Autodesk Inventor part; units mm, degrees
(part 3 of 3)
sketch "Sketch43" plane through (-2.5, -2.5, 2) normal (0, -1, 0) x (1, 0, 0)
  line L0 (109.4941, -32.48) -> (111.9941, -28.1499)
  line L1 (111.9941, -28.1499) -> (116.9941, -28.1499)
  line L2 (116.9941, -28.1499) -> (119.4941, -32.48)
  line L3 (89.4941, -32.48) -> (91.9941, -28.1499) construction
  line L4 (91.9941, -28.1499) -> (96.9941, -28.1499) construction
  line L5 (96.9941, -28.1499) -> (99.4941, -32.48) construction
  line L6 (119.4941, -32.3134) -> (129.4941, -32.3134) construction
  line L7 (119.4941, -19.65) -> (121.9941, -15.3199)
  line L8 (121.9941, -15.3199) -> (126.9941, -15.3199)
  line L9 (126.9941, -23.9801) -> (121.9941, -23.9801)
  line L10 (121.9941, -23.9801) -> (119.4941, -19.65)
  line L11 (109.4941, -6.3326) -> (111.9941, -2.0025)
  line L12 (111.9941, -10.6628) -> (109.4941, -6.3326)
  line L13 (116.9941, -10.6628) -> (111.9941, -10.6628)
  line L14 (111.9941, -2.0025) -> (116.9941, -2.0025)
  line L15 (119.4941, -6.3326) -> (116.9941, -10.6628)
  line L16 (116.9941, -2.0025) -> (119.4941, -6.3326)
  line L17 (96.9941, -10.6628) -> (91.9941, -10.6628)
  line L18 (91.9941, -10.6628) -> (89.4941, -6.3326)
  line L19 (99.4941, -6.3326) -> (96.9941, -10.6628)
  line L20 (89.4941, -6.3326) -> (91.9941, -2.0025)
  line L21 (91.9941, -2.0025) -> (96.9941, -2.0025)
  line L22 (96.9941, -2.0025) -> (99.4941, -6.3326)
  line L23 (99.4941, -19.65) -> (101.9941, -15.3199)
  line L24 (101.9941, -15.3199) -> (106.9941, -15.3199)
  line L25 (106.9941, -15.3199) -> (109.4941, -19.65)
  line L26 (109.4941, -19.65) -> (106.9941, -23.9801)
  line L27 (106.9941, -23.9801) -> (101.9941, -23.9801)
  line L28 (101.9941, -23.9801) -> (99.4941, -19.65)
  line L29 (69.4941, -32.48) -> (71.9941, -28.1499)
  line L30 (71.9941, -28.1499) -> (76.9941, -28.1499)
  line L31 (76.9941, -28.1499) -> (79.4941, -32.48)
  line L32 (49.4941, -32.48) -> (51.9941, -28.1499)
  line L33 (51.9941, -28.1499) -> (56.9941, -28.1499)
  line L34 (56.9941, -28.1499) -> (59.4941, -32.48)
  line L35 (79.4941, -32.48) -> (89.4941, -32.48) construction
  line L36 (79.4941, -19.65) -> (81.9941, -15.3199)
  line L37 (81.9941, -23.9801) -> (79.4941, -19.65)
  line L38 (81.9941, -15.3199) -> (86.9941, -15.3199)
  line L39 (86.9941, -15.3199) -> (89.4941, -19.65)
  line L40 (89.4941, -19.65) -> (86.9941, -23.9801)
  line L41 (86.9941, -23.9801) -> (81.9941, -23.9801)
  line L42 (69.4941, -19.65) -> (66.9941, -23.9801)
  line L43 (76.9941, -10.6628) -> (71.9941, -10.6628)
  line L44 (66.9941, -15.3199) -> (69.4941, -19.65)
  line L45 (66.9941, -23.9801) -> (61.9941, -23.9801)
  line L46 (61.9941, -23.9801) -> (59.4941, -19.65)
  line L47 (59.4941, -19.65) -> (61.9941, -15.3199)
  line L48 (61.9941, -15.3199) -> (66.9941, -15.3199)
  line L49 (71.9941, -10.6628) -> (69.4941, -6.3326)
  line L50 (71.9941, -2.0025) -> (76.9941, -2.0025)
  line L51 (69.4941, -6.3326) -> (71.9941, -2.0025)
  line L52 (76.9941, -2.0025) -> (79.4941, -6.3326)
  line L53 (79.4941, -6.3326) -> (76.9941, -10.6628)
  line L54 (59.4941, -6.3326) -> (56.9941, -10.6628)
  line L55 (51.9941, -2.0025) -> (56.9941, -2.0025)
  line L56 (56.9941, -10.6628) -> (51.9941, -10.6628)
  line L57 (49.4941, -6.3326) -> (51.9941, -2.0025)
  line L58 (51.9941, -10.6628) -> (49.4941, -6.3326)
  line L59 (56.9941, -2.0025) -> (59.4941, -6.3326)
  line L60 (29.4941, -32.48) -> (31.9941, -28.1499)
  line L61 (31.9941, -28.1499) -> (36.9941, -28.1499)
  line L62 (36.9941, -28.1499) -> (39.4941, -32.48)
  line L63 (9.4941, -32.48) -> (11.9941, -28.1499)
  line L64 (11.9941, -28.1499) -> (16.9941, -28.1499)
  line L65 (16.9941, -28.1499) -> (19.4941, -32.48)
  line L66 (39.4941, -32.48) -> (49.4941, -32.48) construction
  line L67 (39.4941, -19.65) -> (41.9941, -15.3199)
  line L68 (41.9941, -23.9801) -> (39.4941, -19.65)
  line L69 (41.9941, -15.3199) -> (46.9941, -15.3199)
  line L70 (46.9941, -15.3199) -> (49.4941, -19.65)
  line L71 (49.4941, -19.65) -> (46.9941, -23.9801)
  line L72 (46.9941, -23.9801) -> (41.9941, -23.9801)
  line L73 (29.4941, -19.65) -> (26.9941, -23.9801)
  line L74 (36.9941, -10.6628) -> (31.9941, -10.6628)
  line L75 (26.9941, -15.3199) -> (29.4941, -19.65)
  line L76 (26.9941, -23.9801) -> (21.9941, -23.9801)
  line L77 (21.9941, -23.9801) -> (19.4941, -19.65)
  line L78 (19.4941, -19.65) -> (21.9941, -15.3199)
  line L79 (21.9941, -15.3199) -> (26.9941, -15.3199)
  line L80 (31.9941, -10.6628) -> (29.4941, -6.3326)
  line L81 (31.9941, -2.0025) -> (36.9941, -2.0025)
  line L82 (29.4941, -6.3326) -> (31.9941, -2.0025)
  line L83 (36.9941, -2.0025) -> (39.4941, -6.3326)
  line L84 (39.4941, -6.3326) -> (36.9941, -10.6628)
  line L85 (19.4941, -6.3326) -> (16.9941, -10.6628)
  line L86 (11.9941, -2.0025) -> (16.9941, -2.0025)
  line L87 (16.9941, -10.6628) -> (11.9941, -10.6628)
  line L88 (9.4941, -6.3326) -> (11.9941, -2.0025)
  line L89 (11.9941, -10.6628) -> (9.4941, -6.3326)
  line L90 (16.9941, -2.0025) -> (19.4941, -6.3326)
  line L91 (-3.7978, -28.1499) -> (-1.2978, -32.48)
  line L92 (-1.2978, -32.48) -> (8.7022, -32.48) construction
  line L93 (1.2022, -15.3199) -> (6.2022, -15.3199)
  line L94 (6.2022, -15.3199) -> (8.7022, -19.65)
  line L95 (8.7022, -19.65) -> (6.2022, -23.9801)
  line L96 (6.2022, -23.9801) -> (1.2022, -23.9801)
  line L97 (-3.7978, -2.0025) -> (-1.2978, -6.3326)
  line L98 (-1.2978, -6.3326) -> (-3.7978, -10.6628)
  line L99 (0, 0) -> (129, 0) construction
  line L100 (129.482, 0) -> (94.272, 0) construction
  line L101 (94.272, 0) -> (94.272, -17.053) construction
  line L102 (127, -2) -> (2, -2) construction
  line L103 (94.272, -2) -> (113.4728, -2) construction
  line L104 (126.9941, -15.3199) -> (127.5487, -15.3199) construction
  line L105 (2, -32.48) -> (127, -32.48) construction
  line L106 (119.4941, -32.48) -> (119.4941, -32.6466) construction
  line L107 (6.8, -32.48) -> (121.5, -32.48) construction
  line L108 (119.4941, -32.48) -> (109.4941, -32.48) construction
  line L109 (119.4941, -32.48) -> (109.4941, -32.48)
  line L110 (99.4941, -32.48) -> (89.4941, -32.48) construction
  line L111 (79.4941, -32.48) -> (69.4941, -32.48)
  line L112 (59.4941, -32.48) -> (49.4941, -32.48)
  line L113 (39.4941, -32.48) -> (29.4941, -32.48)
  line L114 (19.4941, -32.48) -> (9.4941, -32.48)
  line L115 (2, -2) -> (2, -32.48) projected
  line L116 (2, -23.9801) -> (2, -15.3199)
  line L117 (126.9941, -23.9801) -> (126.9941, -15.3199)
  line L118 (127, -23.98) -> (127, -6) projected
  line L119 (51.9941, -28.1499) -> (56.9941, -28.1499)
  line L120 (59.4941, -32.48) -> (56.9941, -28.1499)
  line L121 (51.9941, -28.1499) -> (49.4941, -32.48)
  line L122 (49.4941, -32.48) -> (59.4941, -32.48)
  line L123 (127, -32.48) -> (2, -32.48) construction
  line L124 (89.4941, -32.48) -> (99.4941, -32.48) construction
  line L125 (99.4941, -32.48) -> (96.9941, -28.1499) construction
  line L126 (96.9941, -28.1499) -> (91.9941, -28.1499) construction
  line L127 (89.4941, -32.48) -> (99.4941, -32.48)
  line L128 (99.4941, -32.48) -> (96.9941, -28.1499)
  line L129 (96.9941, -28.1499) -> (91.9941, -28.1499)
  line L130 (91.9941, -28.1499) -> (89.4941, -32.48)
  line L131 (126.9941, -23.9801) -> (121.9941, -23.9801)
  line L132 (126.9941, -15.3199) -> (126.9941, -23.9801)
  line L133 (126.9941, -15.3199) -> (121.9941, -15.3199)
  line L134 (121.9941, -15.3199) -> (119.4941, -19.65)
  line L135 (119.4941, -19.65) -> (121.9941, -23.9801)
  line L136 (144.3219, -16.3384) -> (144.3219, -16.6654)
  line L137 (144.3219, -16.3384) -> (144.6489, -16.3384) construction
  point P0 (2.5, -2)
  point P1 (122.5, -2)
  point P2 (6.5, -2)
  point P3 (2, -14.5)
  point P4 (2, -8.5)
  dimension "d1144" = 34.728
  dimension "d1149" = 0.327
  dimension "d1150" = 90
  constraints: 262 end point, 13 collinear, 7 horizontal, 6 parallel, 5 perpendicular, 3 point on line, 1 vertical
  measures "d1144" distance of L99.end L100.end
  measures "d1149" distance of L136.start L136.end
  measures "d1150" angle of L136 L137
extrude "Extrusion37" cut sketch "Sketch43" against normal blind 2
sketch "Sketch44" plane through (-2.5, 83.5, 2) normal (0, 1, 0) x (1, 0, 0)
  line L0 (16.9941, 2.0025) -> (19.4941, 6.3326) projected
  line L1 (19.4941, 6.3326) -> (16.9941, 10.6628) projected
  line L2 (16.9941, 10.6628) -> (11.9941, 10.6628) projected
  line L3 (11.9941, 10.6628) -> (9.4941, 6.3326) projected
  line L4 (9.4941, 6.3326) -> (11.9941, 2.0025) projected
  line L5 (11.9941, 2.0025) -> (16.9941, 2.0025) projected
  line L6 (39.4941, 6.3326) -> (36.9941, 10.6628) projected
  line L7 (36.9941, 10.6628) -> (31.9941, 10.6628) projected
  line L8 (31.9941, 10.6628) -> (29.4941, 6.3326) projected
  line L9 (29.4941, 6.3326) -> (31.9941, 2.0025) projected
  line L10 (31.9941, 2.0025) -> (36.9941, 2.0025) projected
  line L11 (36.9941, 2.0025) -> (39.4941, 6.3326) projected
  line L12 (56.9941, 2.0025) -> (59.4941, 6.3326) projected
  line L13 (59.4941, 6.3326) -> (56.9941, 10.6628) projected
  line L14 (56.9941, 10.6628) -> (51.9941, 10.6628) projected
  line L15 (51.9941, 10.6628) -> (49.4941, 6.3326) projected
  line L16 (49.4941, 6.3326) -> (51.9941, 2.0025) projected
  line L17 (51.9941, 2.0025) -> (56.9941, 2.0025) projected
  line L18 (79.4941, 6.3326) -> (76.9941, 10.6628) projected
  line L19 (76.9941, 10.6628) -> (71.9941, 10.6628) projected
  line L20 (71.9941, 10.6628) -> (69.4941, 6.3326) projected
  line L21 (69.4941, 6.3326) -> (71.9941, 2.0025) projected
  line L22 (71.9941, 2.0025) -> (76.9941, 2.0025) projected
  line L23 (76.9941, 2.0025) -> (79.4941, 6.3326) projected
  line L24 (119.4941, 6.3326) -> (116.9941, 10.6628) projected
  line L25 (116.9941, 10.6628) -> (111.9941, 10.6628) projected
  line L26 (111.9941, 10.6628) -> (109.4941, 6.3326) projected
  line L27 (109.4941, 6.3326) -> (111.9941, 2.0025) projected
  line L28 (111.9941, 2.0025) -> (116.9941, 2.0025) projected
  line L29 (116.9941, 2.0025) -> (119.4941, 6.3326) projected
  line L30 (126.9941, 23.9801) -> (121.9941, 23.9801) projected
  line L31 (121.9941, 23.9801) -> (119.4941, 19.65) projected
  line L32 (119.4941, 19.65) -> (121.9941, 15.3199) projected
  line L33 (121.9941, 15.3199) -> (126.9941, 15.3199) projected
  line L34 (126.9941, 15.3199) -> (126.9941, 23.9801) projected
  line L35 (96.9941, 28.1499) -> (99.4941, 32.48) projected
  line L36 (99.4941, 32.48) -> (89.4941, 32.48) projected
  line L37 (89.4941, 32.48) -> (91.9941, 28.1499) projected
  line L38 (91.9941, 28.1499) -> (96.9941, 28.1499) projected
  line L39 (11.9941, 28.1499) -> (16.9941, 28.1499) projected
  line L40 (16.9941, 28.1499) -> (19.4941, 32.48) projected
  line L41 (19.4941, 32.48) -> (9.4941, 32.48) projected
  line L42 (9.4941, 32.48) -> (11.9941, 28.1499) projected
  line L43 (79.4941, 32.48) -> (69.4941, 32.48) projected
  line L44 (69.4941, 32.48) -> (71.9941, 28.1499) projected
  line L45 (71.9941, 28.1499) -> (76.9941, 28.1499) projected
  line L46 (76.9941, 28.1499) -> (79.4941, 32.48) projected
  line L47 (119.4941, 32.48) -> (109.4941, 32.48) projected
  line L48 (109.4941, 32.48) -> (111.9941, 28.1499) projected
  line L49 (111.9941, 28.1499) -> (116.9941, 28.1499) projected
  line L50 (116.9941, 28.1499) -> (119.4941, 32.48) projected
  line L51 (39.4941, 32.48) -> (29.4941, 32.48) projected
  line L52 (29.4941, 32.48) -> (31.9941, 28.1499) projected
  line L53 (31.9941, 28.1499) -> (36.9941, 28.1499) projected
  line L54 (36.9941, 28.1499) -> (39.4941, 32.48) projected
  line L55 (51.9941, 28.1499) -> (56.9941, 28.1499) projected
  line L56 (56.9941, 28.1499) -> (59.4941, 32.48) projected
  line L57 (59.4941, 32.48) -> (49.4941, 32.48) projected
  line L58 (49.4941, 32.48) -> (51.9941, 28.1499) projected
  line L59 (2, 23.9801) -> (2, 15.3199) projected
  line L60 (2, 15.3199) -> (6.2022, 15.3199) projected
  line L61 (6.2022, 15.3199) -> (8.7022, 19.65) projected
  line L62 (8.7022, 19.65) -> (6.2022, 23.9801) projected
  line L63 (6.2022, 23.9801) -> (2, 23.9801) projected
  line L64 (101.9941, 15.3199) -> (106.9941, 15.3199) projected
  line L65 (106.9941, 15.3199) -> (109.4941, 19.65) projected
  line L66 (109.4941, 19.65) -> (106.9941, 23.9801) projected
  line L67 (106.9941, 23.9801) -> (101.9941, 23.9801) projected
  line L68 (101.9941, 23.9801) -> (99.4941, 19.65) projected
  line L69 (99.4941, 19.65) -> (101.9941, 15.3199) projected
  line L70 (91.9941, 2.0025) -> (96.9941, 2.0025) projected
  line L71 (96.9941, 2.0025) -> (99.4941, 6.3326) projected
  line L72 (99.4941, 6.3326) -> (96.9941, 10.6628) projected
  line L73 (96.9941, 10.6628) -> (91.9941, 10.6628) projected
  line L74 (91.9941, 10.6628) -> (89.4941, 6.3326) projected
  line L75 (89.4941, 6.3326) -> (91.9941, 2.0025) projected
  line L76 (66.9941, 15.3199) -> (69.4941, 19.65) projected
  line L77 (69.4941, 19.65) -> (66.9941, 23.9801) projected
  line L78 (66.9941, 23.9801) -> (61.9941, 23.9801) projected
  line L79 (61.9941, 23.9801) -> (59.4941, 19.65) projected
  line L80 (59.4941, 19.65) -> (61.9941, 15.3199) projected
  line L81 (61.9941, 15.3199) -> (66.9941, 15.3199) projected
  line L82 (81.9941, 23.9801) -> (79.4941, 19.65) projected
  line L83 (79.4941, 19.65) -> (81.9941, 15.3199) projected
  line L84 (81.9941, 15.3199) -> (86.9941, 15.3199) projected
  line L85 (86.9941, 15.3199) -> (89.4941, 19.65) projected
  line L86 (89.4941, 19.65) -> (86.9941, 23.9801) projected
  line L87 (86.9941, 23.9801) -> (81.9941, 23.9801) projected
  line L88 (26.9941, 15.3199) -> (29.4941, 19.65) projected
  line L89 (29.4941, 19.65) -> (26.9941, 23.9801) projected
  line L90 (26.9941, 23.9801) -> (21.9941, 23.9801) projected
  line L91 (21.9941, 23.9801) -> (19.4941, 19.65) projected
  line L92 (19.4941, 19.65) -> (21.9941, 15.3199) projected
  line L93 (21.9941, 15.3199) -> (26.9941, 15.3199) projected
  line L94 (41.9941, 23.9801) -> (39.4941, 19.65) projected
  line L95 (39.4941, 19.65) -> (41.9941, 15.3199) projected
  line L96 (41.9941, 15.3199) -> (46.9941, 15.3199) projected
  line L97 (46.9941, 15.3199) -> (49.4941, 19.65) projected
  line L98 (49.4941, 19.65) -> (46.9941, 23.9801) projected
  line L99 (46.9941, 23.9801) -> (41.9941, 23.9801) projected
  line L100 (129, 34.48) -> (129, 0) projected
  line L101 (0, 0) -> (129, 0) projected
  line L102 (0, 34.48) -> (0, 0) projected
  line L103 (129, 34.48) -> (0, 34.48) projected
  point P0 (2.5, 2)
extrude "Extrusion38" cut sketch "Sketch44" against normal blind 2 contours L5 L4 L3 L2 L1 L0 | L11 L10 L9 L8 L7 L6 | L29 L28 L27 L26 L25 L24 | L34 L33 L32 L31 L30 | L38 L37 L36 L35 | L42 L41 L40 L39 | L46 L45 L44 L43 | L50 L49 L48 L47 | L54 L53 L52 L51 | L58 L57 L56 L55 | L63 L62 L61 L60 L59 | L69 L68 L67 L66 L65 L64 | L75 L74 L73 L72 L71 L70 | L93 L92 L91 L90 L89 L88 | L99 L98 L97 L96 L95 L94
sketch "Sketch45" plane through (-2.5, -2.5, 2) normal (-1, 0, 0) x (0, 0, 1)
  line L0 (-8.5, 20.7927) -> (-8.5, 19.4927) projected
  line L1 (-8.5, 12.6927) -> (-8.5, 20.7927) projected
  line L2 (-8.5, 13.9927) -> (-8.5, 12.6927) projected
  line L3 (-8.5, 13.9927) -> (-8.5, 19.4927) projected
  line L4 (-22.23, 53.625) -> (-22.23, 74.625) projected
  line L5 (-21.73, 74.625) -> (-21.73, 53.625) projected
  line L6 (-2, 53.625) -> (-2, 53.725)
  line L7 (-21.73, 53.725) -> (-21.73, 53.625)
  line L8 (-21.73, 74.525) -> (-21.73, 74.625)
  line L9 (-8.5, 20.7927) -> (-8.5, 102.544)
  line L10 (-8.5, 20.7927) -> (73.2514, 20.7927) construction
  line L11 (-22.23, 53.625) -> (-8.5, 53.625)
  line L12 (-8.5, 53.625) -> (-8.5, 74.625)
  line L13 (-8.5, 74.625) -> (-22.23, 74.625)
  line L14 (-22.23, 74.625) -> (-22.23, 53.625)
  line L15 (-8.5, 74.525) -> (-21.73, 74.525)
  line L16 (-21.73, 74.525) -> (-21.73, 53.725)
  line L17 (-21.73, 53.725) -> (-8.5, 53.725)
  line L18 (-8.5, 53.725) -> (-8.5, 74.525)
  line L19 (-8.5, 102.544) -> (-40.2369, 102.544)
  line L20 (-40.2369, 102.544) -> (-40.2369, -4.3695)
  line L21 (-40.2369, -4.3695) -> (-8.5, -4.3695)
  line L22 (-8.5, -4.3695) -> (-8.5, 102.544)
  line L23 (-8.5, -4.3695) -> (3.6933, -4.3695)
  line L24 (3.6933, -4.3695) -> (3.6933, 102.544)
  line L25 (3.6933, 102.544) -> (-8.5, 102.544)
  line L26 (-8.5, 102.544) -> (-8.5, -4.3695)
  line L27 (-21.73, 53.725) -> (-8.5, 53.725)
  line L28 (-8.5, 53.725) -> (-8.5, 53.625)
  line L29 (-8.5, 53.625) -> (-21.73, 53.625)
  line L30 (-21.73, 53.625) -> (-21.73, 53.725)
  line L31 (-21.73, 74.525) -> (-8.5, 74.525)
  line L32 (-8.5, 74.525) -> (-8.5, 74.625)
  line L33 (-8.5, 74.625) -> (-21.73, 74.625)
  line L34 (-21.73, 74.625) -> (-21.73, 74.525)
  line L35 (-21.73, 74.525) -> (-8.5, 74.525)
  line L36 (-8.5, 74.525) -> (-8.5, 53.725)
  line L37 (-8.5, 53.725) -> (-21.73, 53.725)
  line L38 (-21.73, 53.725) -> (-21.73, 74.525)
  point P0 (-2, 2.5)
  point P1 (-2, 74.525)
  dimension "d1156" = 0.1
  dimension "d1158" = 90
  constraints: 66 end point, 15 parallel, 8 horizontal, 8 perpendicular, 4 point on line
  measures "d1156" distance of L6.end L6.start
  measures "d1158" angle of L10 L9
extrude "Extrusion39" cut sketch "Sketch45" against normal blind 150 contours L0 L1 L22 L21 L20 L19 L9 L13 L4 L11 | L11 L5 L17 L9 | L15 L5 L13 L9
sketch "Sketch50" plane through (0, 0, 0) normal (0, 0, 1) x (1, 0, 0)
  circle A0 centre (122.25, 79.25) radius 1.35
  line L0 (121, 77) -> (124.5, 77)
  line L1 (124.5, 77) -> (124.5, 81.5)
  line L2 (124.5, 81.5) -> (120, 81.5)
  line L3 (120, 81.5) -> (120, 78)
  line L4 (120, 78) -> (121, 77)
  circle A1 centre (122.25, 1.75) radius 1.35
  line L5 (124.5, 4) -> (120, 4)
  line L6 (120, 4) -> (120, -0.5)
  line L7 (120, -0.5) -> (124.5, -0.5)
  line L8 (124.5, -0.5) -> (124.5, 4)
  circle A2 centre (1.75, 1.75) radius 1.35
  arc A3 (3.2216, 4) -> (4, 2.8097) centre (6.05, 5) ccw
  line L9 (3.2216, 4) -> (-0.5, 4)
  line L10 (-0.5, 4) -> (-0.5, -0.5)
  line L11 (-0.5, -0.5) -> (4, -0.5)
  line L12 (4, -0.5) -> (4, 2.8097)
  circle A4 centre (1.75, 79.25) radius 1.35
  line L13 (-0.5, 77) -> (4, 77)
  line L14 (4, 77) -> (4, 81.5)
  line L15 (4, 81.5) -> (-0.5, 81.5)
  line L16 (-0.5, 81.5) -> (-0.5, 77)
  point P0 (0, 0)
  point P1 (0, 0)
  constraints: 34 end point, 5 centre point, 2 point on circle
sketch "Sketch51" plane through (0, 0, -6.5) normal (0, 0, -1) x (-1, 0, 0)
  line L0 (-4, 81.5) -> (-4, 77) projected
  line L1 (-4, 77) -> (0.5, 77)
  line L2 (0.5, 77) -> (0.5, 81.5)
  line L3 (0.5, 81.5) -> (-4, 81.5)
  line L4 (-4, 81.5) -> (-4, 77)
  line L5 (0.5, 4) -> (-3.2216, 4) projected
  line L6 (-8.2455, -0.5) -> (-4, -0.5) projected
  line L7 (0.5, 4) -> (-4, 4)
  line L8 (-4, 4) -> (-4, -0.5)
  line L9 (-4, -0.5) -> (0.5, -0.5)
  line L10 (0.5, -0.5) -> (0.5, 4)
  line L11 (-81, 81.5) -> (-120, 81.5) projected
  line L12 (-120, 81.5) -> (-124.5, 81.5)
  line L13 (-124.5, 81.5) -> (-124.5, 77)
  line L14 (-124.5, 77) -> (-120, 77)
  line L15 (-120, 77) -> (-120, 81.5)
  line L16 (-124.5, 4) -> (-120, 4) projected
  line L17 (-120, 4) -> (-124.5, 4)
  line L18 (-124.5, 4) -> (-124.5, -0.5)
  line L19 (-124.5, -0.5) -> (-120, -0.5)
  line L20 (-120, -0.5) -> (-120, 4)
  point P0 (0, 0)
  dimension "d1212" = 4.5
  dimension "d1213" = 4.5
  dimension "d1214" = 4.5
  dimension "d1215" = 4.5
  dimension "d1216" = 4.5
  dimension "d1217" = 4.5
  dimension "d1218" = 4.5
  dimension "d1219" = 4.5
  constraints: 32 end point, 8 parallel, 4 horizontal, 4 perpendicular
  measures "d1212" distance of L3.end L2.end
  measures "d1213" distance of L2.end L1.end
  measures "d1214" distance of L9.end L6.end
  measures "d1215" distance of L6.end L7.end
  measures "d1216" distance of L14.end L13.end
  measures "d1217" distance of L13.end L12.end
  measures "d1218" distance of L19.end L18.end
  measures "d1219" distance of L18.end L17.end
extrude "Extrusion43" cut sketch "Sketch51" against normal blind 3
equation "\"d67\" = d68"
equation "\"d69\" = d68"
equation "\"d70\" = d68"
equation "\"d112\" = d68"
equation "\"d113\" = d68"
equation "\"d114\" = d68"
body "Solid1"
